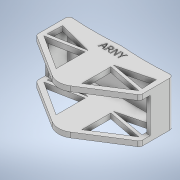
# Autodesk Inventor part: Torso
Saved by Autodesk Inventor 2022 (Build 260153000, 153)
## iProperties
Created: 2022-04-29
Part Number: Torso
Material: Generic
Document SubType Name: Modeling
Designer: kajve
Density: 1 g/cm^3
Appearance: Default
Author: kajve
Autodesk Inventor part; units mm, degrees
ref_plane "YZ Plane" through (0, 0, 0) normal (1, 0, 0) x (0, 1, 0)
ref_plane "XZ Plane" through (0, 0, 0) normal (0, 1, 0) x (-1, 0, 0)
ref_plane "XY Plane" through (0, 0, 0) normal (0, 0, 1) x (1, 0, 0)
sketch "Sketch1" plane through (0, 0, 0) normal (0, 0, 1) x (1, 0, 0)
  line L0 (0, 0) -> (307.0476, 0)
  line L1 (307.0476, 0) -> (307.0476, 132.8995)
  line L2 (307.0476, 132.8995) -> (0, 132.8995)
  line L3 (0, 132.8995) -> (0, 0)
  dimension "d0" = 307.0476
  dimension "d1" = 132.8995
  constraints: 8 end point, 2 parallel, 1 horizontal, 1 perpendicular
  measures "d0" distance of L1.end L2.end
  measures "d1" distance of L0.end L1.end
extrude "Extrusion1" add sketch "Sketch1" along normal blind 250
sketch "Sketch2" plane through (0, 132.8995, 0) normal (0, 1, 0) x (1, 0, 0)
  line L0 (0, 0) -> (0, -250) projected
  line L1 (307.0476, -250) -> (0, -250) projected
  line L2 (307.0476, 0) -> (307.0476, -250) projected
  line L3 (0, -194.0642) -> (307.0476, -194.0642)
  line L4 (307.0476, -194.0642) -> (307.0476, -250)
  line L5 (307.0476, -250) -> (0, -250)
  line L6 (0, -250) -> (0, -194.0642)
  constraints: 8 end point, 2 parallel, 1 horizontal, 1 perpendicular, 1 point on line
extrude "Extrusion2" cut sketch "Sketch2" against normal blind 250
sketch "Sketch3" plane through (0, 132.8995, 0) normal (0, 1, 0) x (1, 0, 0)
  line L0 (0, -194.0642) -> (307.0476, -194.0642) projected
  line L1 (307.0476, 0) -> (307.0476, -194.0642) projected
  line L2 (0, 0) -> (0, -194.0642) projected
  line L3 (0, -97.0321) -> (126.8105, -177.1805)
  line L4 (180.2372, -177.1805) -> (307.0476, -97.0321)
  arc A0 (126.8105, -177.1805) -> (180.2372, -177.1805) centre (153.5238, -134.9147) ccw
  point P0 (153.5238, -194.0642)
  dimension "d8" = 50
  constraints: 4 end point, 3 midpoint, 2 point on circle, 2 point on line, 2 tangent, 1 centre point
  measures "d8" radius of A0
extrude "Extrusion3" cut sketch "Sketch3" against normal blind 250
sketch "Sketch4" plane through (0, 0, 0) normal (-1, 0, 0) x (0, 0, 1)
  line L0 (184.9147, 0) -> (184.9147, 132.8995) projected
  line L1 (15, 15) -> (184.9147, 15)
  line L2 (184.9147, 15) -> (184.9147, 117.9)
  line L3 (184.9147, 117.9) -> (15, 117.9)
  line L4 (15, 117.9) -> (15, 15)
  dimension "d9" = 102.9
  constraints: 8 end point, 2 parallel, 1 horizontal, 1 perpendicular, 1 point on line
  measures "d9" distance of L2.end L1.end
extrude "Extrusion4" cut sketch "Sketch4" against normal through all
sketch "Sketch5" plane through (0, 132.8995, 0) normal (0, 1, 0) x (1, 0, 0)
  line L0 (180.2372, -177.1805) -> (307.0476, -97.0321) projected
  line L1 (307.0476, 0) -> (307.0476, -97.0321) projected
  line L2 (307.0476, 0) -> (0, 0) projected
  line L3 (0, 0) -> (0, -97.0321) projected
  line L4 (0, -97.0321) -> (126.8105, -177.1805) projected
  arc A0 (126.8105, -177.1805) -> (180.2372, -177.1805) centre (153.5238, -134.9147) ccw projected
sketch "Sketch6" plane through (0, 132.8995, 0) normal (0, 1, 0) x (1, 0, 0)
  arc A0 (126.8105, -177.1805) -> (180.2372, -177.1805) centre (153.5238, -134.9147) ccw projected
  line L0 (119.161, -15.0078) -> (129.54, -15.0078) construction
  line L1 (129.54, -15.0078) -> (129.54, -18.0558) construction
  line L2 (129.54, -18.0558) -> (119.161, -18.0558) construction
  line L3 (119.161, -18.0558) -> (119.161, -15.0078) construction
  line L4 (0, 0) -> (307.0476, 0) construction
  line L5 (153.5238, 0) -> (153.5238, -184.9147) construction
  arc A1 (126.8105, -177.1805) -> (180.2372, -177.1805) centre (153.5238, -134.9147) ccw construction
  line L6 (119.0313, -35.0078) -> (125.7736, -15.0078)
  line L7 (125.7736, -15.0078) -> (129.0475, -15.0078)
  line L8 (129.0475, -15.0078) -> (135.7898, -35.0078)
  line L9 (135.7898, -35.0078) -> (132.9859, -35.0078)
  line L10 (132.9859, -35.0078) -> (131.1707, -29.4163)
  line L11 (131.1707, -29.4163) -> (123.537, -29.4163)
  line L12 (123.537, -29.4163) -> (121.7218, -35.0078)
  line L13 (121.7218, -35.0078) -> (119.0313, -35.0078)
  line L14 (130.4414, -27.1472) -> (127.3457, -17.7307)
  line L15 (127.3457, -17.7307) -> (124.2663, -27.1472)
  line L16 (124.2663, -27.1472) -> (130.4414, -27.1472)
  line L17 (153.1642, -35.0078) -> (149.712, -35.0078)
  line L18 (149.712, -35.0078) -> (143.3911, -27.05)
  line L19 (143.3911, -27.05) -> (140.3441, -27.05)
  line L20 (140.3441, -27.05) -> (140.3441, -35.0078)
  line L21 (140.3441, -35.0078) -> (137.6861, -35.0078)
  line L22 (137.6861, -35.0078) -> (137.6861, -15.0078)
  line L23 (137.6861, -15.0078) -> (142.8401, -15.0078)
  spline S0 degree 2 poles (142.8401, -15.0078) (144.5581, -15.0078) (146.8757, -15.3806) (147.9292, -16.0613) knots 0 0 0 1 2 2 2
  spline S1 degree 2 poles (147.9292, -16.0613) (148.9827, -16.742) (150.1983, -18.8652) (150.1983, -20.4373) knots 0 0 0 1 2 2 2
  spline S2 degree 2 poles (150.1983, -20.4373) (150.1983, -22.6253) (147.9616, -25.5913) (146.0491, -26.3044) knots 0 0 0 1 2 2 2
  line L24 (146.0491, -26.3044) -> (153.1642, -35.0078)
  spline S3 degree 2 poles (147.4268, -20.648) (147.4268, -19.7728) (146.8109, -18.4276) (146.1626, -17.99) knots 0 0 0 1 2 2 2
  spline S4 degree 2 poles (146.1626, -17.99) (145.5953, -17.6172) (144.088, -17.3093) (142.9859, -17.3093) knots 0 0 0 1 2 2 2
  line L25 (142.9859, -17.3093) -> (140.3441, -17.3093)
  line L26 (140.3441, -17.3093) -> (140.3441, -24.8296)
  line L27 (140.3441, -24.8296) -> (142.678, -24.8296)
  spline S5 degree 2 poles (142.678, -24.8296) (143.8287, -24.8296) (145.6602, -24.4244) (146.2923, -23.7923) knots 0 0 0 1 2 2 2
  spline S6 degree 2 poles (146.2923, -23.7923) (146.8757, -23.2412) (147.4268, -21.6853) (147.4268, -20.648) knots 0 0 0 1 2 2 2
  line L28 (169.0637, -35.0078) -> (166.0816, -35.0078)
  line L29 (166.0816, -35.0078) -> (157.2323, -17.7631)
  line L30 (157.2323, -17.7631) -> (157.2323, -35.0078)
  line L31 (157.2323, -35.0078) -> (154.7525, -35.0078)
  line L32 (154.7525, -35.0078) -> (154.7525, -15.0078)
  line L33 (154.7525, -15.0078) -> (158.5289, -15.0078)
  line L34 (158.5289, -15.0078) -> (166.584, -30.8425)
  line L35 (166.584, -30.8425) -> (166.584, -15.0078)
  line L36 (166.584, -15.0078) -> (169.0637, -15.0078)
  line L37 (169.0637, -15.0078) -> (169.0637, -35.0078)
  line L38 (187.1188, -15.0078) -> (180.3603, -26.1586)
  line L39 (180.3603, -26.1586) -> (180.3603, -35.0078)
  line L40 (180.3603, -35.0078) -> (177.7023, -35.0078)
  line L41 (177.7023, -35.0078) -> (177.7023, -26.4341)
  line L42 (177.7023, -26.4341) -> (170.9438, -15.0078)
  line L43 (170.9438, -15.0078) -> (173.8936, -15.0078)
  line L44 (173.8936, -15.0078) -> (179.0475, -23.8085)
  line L45 (179.0475, -23.8085) -> (184.2987, -15.0078)
  line L46 (184.2987, -15.0078) -> (187.1188, -15.0078)
  constraints: 2 end point, 2 point on circle, 1 midpoint, 2 other
extrude "Extrusion5" cut sketch "Sketch6" against normal blind 3
sketch "Sketch7" plane through (0, 132.8995, 0) normal (0, 1, 0) x (1, 0, 0)
  arc A0 (126.8105, -177.1805) -> (180.2372, -177.1805) centre (153.5238, -134.9147) ccw projected
  line L0 (13.5639, -88.7516) -> (115.7433, -154.4248)
  line L1 (115.7433, -154.4248) -> (115.7433, -68.9852)
  line L2 (115.7433, -68.9852) -> (13.5639, -88.7516)
  line L3 (0, 0) -> (307.0476, 0) construction
  line L4 (153.5238, 0) -> (153.5238, -184.9147) construction
  arc A1 (126.8105, -177.1805) -> (180.2372, -177.1805) centre (153.5238, -134.9147) ccw construction
  line L5 (293.4838, -88.7516) -> (191.3043, -154.4248)
  line L6 (191.3043, -154.4248) -> (191.3043, -68.9852)
  line L7 (191.3043, -68.9852) -> (293.4838, -88.7516)
  line L8 (13.5639, -88.7516) -> (293.4838, -88.7516) construction
  line L9 (191.3043, -154.4248) -> (115.7433, -154.4248) construction
  line L10 (115.7433, -68.9852) -> (191.3043, -68.9852) construction
  line L11 (307.0476, -97.0321) -> (180.2372, -177.1805) construction
  constraints: 20 end point, 4 symmetric about line, 2 parallel, 2 point on circle, 1 horizontal, 1 midpoint, 1 vertical
extrude "Extrusion6" cut sketch "Sketch7" against normal through all
sketch "Sketch8" plane through (0, 132.8995, 0) normal (0, 1, 0) x (1, 0, 0)
  line L0 (307.0476, 0) -> (0, 0) projected
  line L1 (115.7433, -60.8817) -> (13.5639, -78.8684)
  line L2 (13.5639, -78.8684) -> (15.6629, -35.0078)
  line L3 (15.6629, -35.0078) -> (115.7433, -60.8817)
  line L4 (153.5238, 0) -> (153.5238, -184.9147) construction
  arc A0 (126.8105, -177.1805) -> (180.2372, -177.1805) centre (153.5238, -134.9147) ccw construction
  line L5 (191.3043, -60.8817) -> (293.4838, -78.8684)
  line L6 (293.4838, -78.8684) -> (291.3847, -35.0078)
  line L7 (291.3847, -35.0078) -> (191.3043, -60.8817)
  constraints: 14 end point, 3 symmetric about line, 1 midpoint, 1 point on circle
extrude "Extrusion7" cut sketch "Sketch8" against normal through all
sketch "Sketch9" plane through (0, 132.8995, 0) normal (0, 1, 0) x (1, 0, 0)
  line L0 (307.0476, 0) -> (0, 0) projected
  arc A0 (126.8105, -177.1805) -> (180.2372, -177.1805) centre (153.5238, -134.9147) ccw projected
  arc A1 (0, 0) -> (153.5238, 0) centre (76.7619, 882.9835) ccw
  line L1 (153.5238, 0) -> (153.5238, -184.9147) construction
  arc A2 (126.8105, -177.1805) -> (180.2372, -177.1805) centre (153.5238, -134.9147) ccw construction
  arc A3 (153.5238, 0) -> (307.0476, 0) centre (230.2857, 882.9835) ccw
  constraints: 6 point on circle, 2 centre point, 2 end point, 1 midpoint, 1 symmetric about line, 1 other
extrude "Extrusion8" cut sketch "Sketch9" against normal through all
fillet "Fillet1" radius 10 6 edges at (0, 66.4498, 0) (307.0476, 66.4498, 0) (307.0476, 125.3998, 97.0321) (307.0476, 7.5, 97.0321) (0, 125.3998, 97.0321) (0, 7.5, 97.0321)
sketch "Sketch10" plane through (307.0476, 15, 15) normal (1, 0, 0) x (0, 0, -1)
  line L0 (-76.5225, 102.9) -> (0, 102.9) projected
  line L1 (0, 102.9) -> (0, 0) projected
  line L2 (0, 0) -> (-76.5225, 0) projected
  line L3 (0, 0) -> (0, 102.9) projected
  line L4 (-73.7516, 0) -> (-53.9852, 0) projected
  line L5 (0, 102.9) -> (-53.9852, 102.9)
  line L6 (-53.9852, 102.9) -> (-53.9852, 0)
  line L7 (-53.9852, 0) -> (0, 0)
  line L8 (0, 0) -> (0, 102.9)
  point P0 (15, -15)
  constraints: 8 end point, 2 parallel, 1 horizontal, 1 perpendicular
extrude "Extrusion9" add sketch "Sketch10" against normal blind 10
sketch "Sketch11" plane through (0, 15, 15) normal (-1, 0, 0) x (0, 0, 1)
  line L0 (76.5225, 0) -> (0, 0) projected
  line L1 (0, 0) -> (0, 102.9) projected
  line L2 (0, 102.9) -> (76.5225, 102.9) projected
  line L3 (53.9852, 0) -> (0, 0) projected
  line L4 (63.8684, 102.9) -> (45.8817, 102.9) projected
  line L5 (0, 0) -> (54.875, 0)
  line L6 (54.875, 0) -> (54.875, 102.9)
  line L7 (54.875, 102.9) -> (0, 102.9)
  line L8 (0, 102.9) -> (0, 0)
  point P0 (-15, -15)
  constraints: 8 end point, 2 parallel, 1 horizontal, 1 midpoint, 1 perpendicular
extrude "Extrusion10" add sketch "Sketch11" against normal blind 10
body "Solid1"
